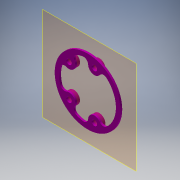
# Autodesk Inventor part: Ring Front
Saved by Autodesk Inventor 2017 (Build 210142000, 142)
## iProperties
Created: 2016-12-22
Part Number: Ring Front
Material: Generic
Document SubType Name: Modeling
Designer: PLTW
Density: 1 g/cm^3
Appearance: Magenta
Author: PLTW
Autodesk Inventor part; units mm, degrees
ref_plane "YZ Plane" through (0, 0, 0) normal (1, 0, 0) x (0, 1, 0)
ref_plane "XZ Plane" through (0, 0, 0) normal (0, 1, 0) x (-1, 0, 0)
ref_plane "XY Plane" through (0, 0, 0) normal (0, 0, 1) x (1, 0, 0)
ref_plane "Work Plane1" through (0, 0, 0) normal (0, 0, 1) x (1, 0, 0)
sketch "Sketch1" plane through (0, 0, 0) normal (0, 0, 1) x (1, 0, 0)
  line L0 (-8.3321, -22.7734) -> (-9.471, -25.3313) construction
  line L1 (-9.471, -25.3313) -> (-12.4875, -23.9883) construction
  line L2 (-12.4875, -23.9883) -> (-11.3486, -21.4303) construction
  line L3 (-11.3486, -21.4303) -> (-8.3321, -22.7734) construction
  line L4 (-16.8745, -17.4155) -> (-18.9553, -19.2891) construction
  line L5 (-18.9553, -19.2891) -> (-21.1648, -16.8352) construction
  line L6 (-21.1648, -16.8352) -> (-19.084, -14.9617) construction
  line L7 (-19.084, -14.9617) -> (-16.8745, -17.4155) construction
  line L8 (-22.4992, -9.0464) -> (-25.1622, -9.9116) construction
  line L9 (-25.1622, -9.9116) -> (-26.1825, -6.7713) construction
  line L10 (-26.1825, -6.7713) -> (-23.5196, -5.906) construction
  line L11 (-23.5196, -5.906) -> (-22.4992, -9.0464) construction
  line L12 (-24.2335, 0.887) -> (-27.0182, 1.1796) construction
  line L13 (-27.0182, 1.1796) -> (-26.6731, 4.4635) construction
  line L14 (-26.6731, 4.4635) -> (-23.8884, 4.1709) construction
  line L15 (-23.8884, 4.1709) -> (-24.2335, 0.887) construction
  line L16 (-21.7777, 10.6669) -> (-24.2026, 12.0669) construction
  line L17 (-24.2026, 12.0669) -> (-22.5516, 14.9266) construction
  line L18 (-22.5516, 14.9266) -> (-20.1267, 13.5266) construction
  line L19 (-20.1267, 13.5266) -> (-21.7777, 10.6669) construction
  line L20 (-15.5563, 18.6025) -> (-17.2021, 20.8678) construction
  line L21 (-17.2021, 20.8678) -> (-14.5307, 22.8086) construction
  line L22 (-14.5307, 22.8086) -> (-12.8849, 20.5434) construction
  line L23 (-12.8849, 20.5434) -> (-15.5563, 18.6025) construction
  line L24 (-6.645, 23.3216) -> (-7.2272, 26.0604) construction
  line L25 (-7.2272, 26.0604) -> (-3.9973, 26.7469) construction
  line L26 (-3.9973, 26.7469) -> (-3.4152, 24.0081) construction
  line L27 (-3.4152, 24.0081) -> (-6.645, 23.3216) construction
  line L28 (3.4152, 24.0081) -> (3.9973, 26.7469) construction
  line L29 (3.9973, 26.7469) -> (7.2272, 26.0604) construction
  line L30 (7.2272, 26.0604) -> (6.645, 23.3216) construction
  line L31 (6.645, 23.3216) -> (3.4152, 24.0081) construction
  line L32 (12.8849, 20.5434) -> (14.5307, 22.8086) construction
  line L33 (14.5307, 22.8086) -> (17.2021, 20.8678) construction
  line L34 (17.2021, 20.8678) -> (15.5563, 18.6025) construction
  line L35 (15.5563, 18.6025) -> (12.8849, 20.5434) construction
  line L36 (20.1267, 13.5266) -> (22.5516, 14.9266) construction
  line L37 (22.5516, 14.9266) -> (24.2026, 12.0669) construction
  line L38 (24.2026, 12.0669) -> (21.7777, 10.6669) construction
  line L39 (21.7777, 10.6669) -> (20.1267, 13.5266) construction
  line L40 (23.8884, 4.1709) -> (26.6731, 4.4635) construction
  line L41 (26.6731, 4.4635) -> (27.0182, 1.1796) construction
  line L42 (27.0182, 1.1796) -> (24.2335, 0.887) construction
  line L43 (24.2335, 0.887) -> (23.8884, 4.1709) construction
  line L44 (23.5196, -5.906) -> (26.1825, -6.7713) construction
  line L45 (26.1825, -6.7713) -> (25.1622, -9.9116) construction
  line L46 (25.1622, -9.9116) -> (22.4992, -9.0464) construction
  line L47 (22.4992, -9.0464) -> (23.5196, -5.906) construction
  line L48 (19.084, -14.9617) -> (21.1648, -16.8352) construction
  line L49 (21.1648, -16.8352) -> (18.9553, -19.2891) construction
  line L50 (18.9553, -19.2891) -> (16.8745, -17.4155) construction
  line L51 (16.8745, -17.4155) -> (19.084, -14.9617) construction
  line L52 (11.3486, -21.4303) -> (12.4875, -23.9883) construction
  line L53 (12.4875, -23.9883) -> (9.471, -25.3313) construction
  line L54 (9.471, -25.3313) -> (8.3321, -22.7734) construction
  line L55 (8.3321, -22.7734) -> (11.3486, -21.4303) construction
  line L56 (1.651, -24.1935) -> (1.651, -26.9935) construction
  line L57 (1.651, -26.9935) -> (-1.651, -26.9935) construction
  line L58 (-1.651, -26.9935) -> (-1.651, -24.1935) construction
  line L59 (-1.651, -24.1935) -> (1.651, -24.1935) construction
  circle A0 centre (0, 0) radius 21.9075 construction
  circle A1 centre (0, 0) radius 29.972 construction
  line L60 (-34.3408, 32.385) -> (-34.3408, -32.385) construction
  line L61 (-34.3408, -32.385) -> (15.5702, -32.385) construction
  line L62 (15.5702, -32.385) -> (15.5702, 32.385) construction
  line L63 (15.5702, 32.385) -> (-34.3408, 32.385) construction
  circle A2 centre (-26.2128, 23.749) radius 1.524 construction
  circle A3 centre (6.9342, -23.749) radius 1.524 construction
  line L64 (-2.9845, -10.0203) -> (-2.9845, -9.271) construction
  line L65 (-2.9845, -9.271) -> (-9.271, -9.271) construction
  line L66 (-9.271, -9.271) -> (-9.271, 9.271) construction
  line L67 (-9.271, 9.271) -> (-2.9845, 9.271) construction
  line L68 (-2.9845, 9.271) -> (-2.9845, 10.0203) construction
  arc A4 (2.9845, 10.0203) -> (-2.9845, 10.0203) centre (0, 10.0203) ccw construction
  line L69 (2.9845, 10.0203) -> (2.9845, 9.271) construction
  line L70 (2.9845, 9.271) -> (9.271, 9.271) construction
  line L71 (9.271, 9.271) -> (9.271, -9.271) construction
  line L72 (9.271, -9.271) -> (2.9845, -9.271) construction
  line L73 (2.9845, -9.271) -> (2.9845, -10.0203) construction
  arc A5 (-2.9845, -10.0203) -> (2.9845, -10.0203) centre (0, -10.0203) ccw construction
  circle A6 centre (4.826, 16.7824) radius 1.905
  circle A7 centre (4.826, -16.7824) radius 1.905
  circle A8 centre (-13.081, 11.5683) radius 1.905
  circle A9 centre (-13.081, -11.5683) radius 1.905
  circle A10 centre (0, 0) radius 23.1775
  arc A11 (1.6885, 19.9311) -> (9.1568, 17.7835) centre (4.826, 16.7824) ccw
  arc A12 (9.1568, -17.7835) -> (1.6885, -19.9311) centre (4.826, -16.7824) ccw
  arc A13 (-12.1243, -15.9092) -> (-17.2723, -10.088) centre (-13.081, -11.5683) ccw
  arc A14 (-17.2723, 10.088) -> (-12.1243, 15.9092) centre (-13.081, 11.5683) ccw
  arc A15 (-12.1243, -15.9092) -> (1.6885, -19.9311) centre (0, 0) ccw
  arc A16 (-17.2723, 10.088) -> (-17.2723, -10.088) centre (0, 0) ccw
  arc A17 (9.1568, -17.7835) -> (9.1568, 17.7835) centre (0, 0) ccw
  arc A18 (1.6885, 19.9311) -> (-12.1243, 15.9092) centre (0, 0) ccw
  dimension "d0" = 2.54
  dimension "d1" = 2.54
  dimension "d2" = 2.54
  dimension "d3" = 2.54
  dimension "d4" = 3.81
  dimension "d5" = 2.54
  dimension "d6" = 3.81
  dimension "d7" = 1.27
  dimension "d9" = 2.54
  dimension "d10" = 3.175
  dimension "d11" = 3.175
  dimension "d12" = 3.175
  dimension "d13" = 3.175
  constraints: 16 point on circle, 13 centre point, 6 coincident, 6 equal radius, 2 vertical alignment
  measures "d4" diameter of A6
  measures "d5" distance edge to line of A6 L71
  measures "d6" horizontal distance of L66.end A8.centre
  measures "d7" radial gap between concentric circles of A0 A10
  measures "d9" radial gap between concentric circles of A6 A11
  measures "d10" radial gap between concentric circles of A10 A17
  measures "d11" radial gap between concentric circles of A18 A10
  measures "d12" radial gap between concentric circles of A10 A16
  measures "d13" radial gap between concentric circles of A10 A15
extrude "Extrusion1" add sketch "Sketch1" along normal blind 1.27
fillet "Fillet1" radius 3.175 8 edges at (9.1568, 17.7835, 0.635) (1.6885, 19.9311, 0.635) (-12.1243, 15.9092, 0.635) (-17.2723, 10.088, 0.635) (9.1568, -17.7835, 0.635) (1.6885, -19.9311, 0.635) (-12.1243, -15.9092, 0.635) (-17.2723, -10.088, 0.635)
sketch "Sketch2" plane through (0, 0, 0) normal (0, 0, -1) x (-1, 0, 0)
  circle A0 centre (13.081, -11.5683) radius 1.905 projected
  circle A1 centre (13.081, 11.5683) radius 1.905 projected
  circle A2 centre (-4.826, -16.7824) radius 1.905 projected
  circle A3 centre (-4.826, 16.7824) radius 1.905 projected
  circle A4 centre (-4.826, -16.7824) radius 4.318
  circle A5 centre (-4.826, 16.7824) radius 1.905 projected
  circle A6 centre (-4.826, 16.7824) radius 4.318
  circle A7 centre (13.081, -11.5683) radius 1.905 projected
  circle A8 centre (13.081, -11.5683) radius 4.318
  circle A9 centre (13.081, 11.5683) radius 4.318
  circle A10 centre (0, 0) radius 21.9075 construction
  dimension "d17" = 0.127
  constraints: 4 centre point, 3 coincident, 3 equal radius, 1 concentric
extrude "Extrusion2" add sketch "Sketch2" along normal blind 2.159
equation "\"d1\" = d0"
equation "\"d2\" = d1"
equation "\"d3\" = d0"
body "Solid1"
